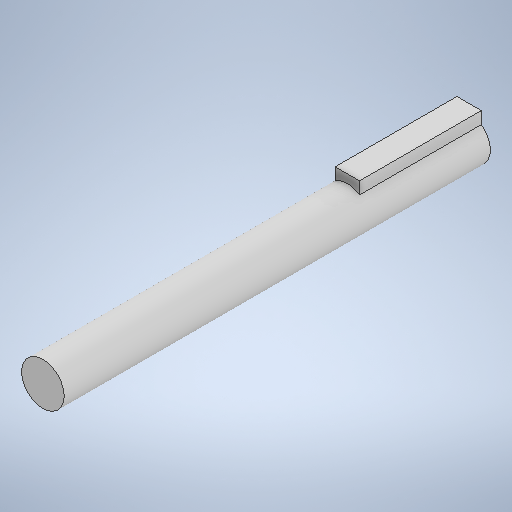
# Autodesk Inventor part: shaft1
Saved by Autodesk Inventor 2025 (Build 290162010, 162A)
## iProperties
Created: 2024-07-26
Part Number: shaft1
Material: Generic
Document SubType Name: Modeling
Designer: saees
Density: 1 g/cm^3
Appearance: Default
Author: saees
Autodesk Inventor part; units mm, degrees
ref_plane "YZ Plane" through (0, 0, 0) normal (1, 0, 0) x (0, 1, 0)
ref_plane "XZ Plane" through (0, 0, 0) normal (0, 1, 0) x (-1, 0, 0)
ref_plane "XY Plane" through (0, 0, 0) normal (0, 0, 1) x (1, 0, 0)
sketch "Sketch1" plane through (0, 0, 0) normal (0, 0, 1) x (1, 0, 0)
  circle A0 centre (0, 0) radius 3.5
  dimension "d0" = 7
  constraints: 1 centre point, 1 coincident
  measures "d0" diameter of A0
extrude "Extrusion1" add sketch "Sketch1" along normal blind 70
sketch "Sketch2" plane through (0, 0, 0) normal (0, 0, -1) x (-1, 0, 0)
  circle A0 centre (0, 0) radius 3.5 projected
  line L0 (-2, 2.8723) -> (-2, 4.8723)
  line L1 (-2, 4.8723) -> (2, 4.8723)
  line L2 (2, 4.8723) -> (2, 2.8723)
  arc A1 (2, 2.8723) -> (-2, 2.8723) centre (0, 0) ccw
  point P0 (0, 4.8723)
  dimension "d3" = 4
  dimension "d4" = 2
  constraints: 6 end point, 5 point on circle, 2 concentric, 2 perpendicular, 1 centre point, 1 midpoint, 1 vertical, 1 vertical alignment
  measures "d3" distance of L0.end L1.end
  measures "d4" distance of L1.end L2.end
extrude "Extrusion2" add sketch "Sketch2" against normal blind 20 contours A0 L0 L1 L2
body "Solid1"
